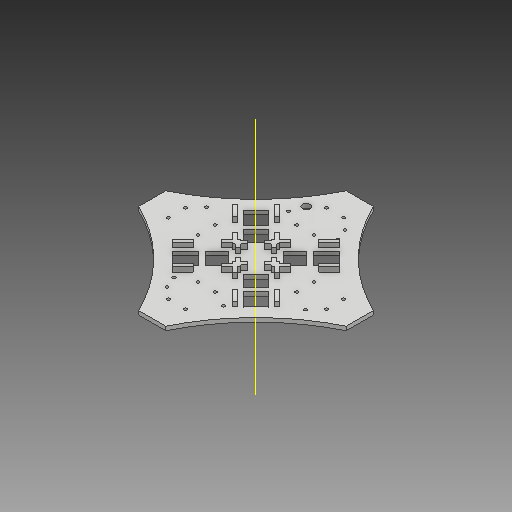
# Autodesk Inventor part: grundplatte_unten
Saved by Autodesk Inventor 2019 (Build 230136000, 136)
## iProperties
Created: 2018-07-23
Part Number: grundplatte_unten
Material: Generisch
Document SubType Name: Modeling
Designer: juliu
Density: 1 g/cm^3
Appearance: Vorgabe
Author: juliu
Autodesk Inventor part; units mm, degrees
ref_plane "YZ Plane" through (0, 0, 0) normal (1, 0, 0) x (0, 1, 0)
ref_plane "XZ Plane" through (0, 0, 0) normal (0, 1, 0) x (-1, 0, 0)
ref_plane "XY Plane" through (0, 0, 0) normal (0, 0, 1) x (1, 0, 0)
sketch "Skizze2" plane through (0, 0, 0) normal (0, 0, 1) x (1, 0, 0)
  line L0 (-268.185, 0) -> (268.185, 0)
  line L1 (0, -270.5283) -> (0, 270.5283) projected
  line L2 (-13.75, 105) -> (13.75, 105)
  line L3 (105, 13.75) -> (105, -13.75)
  line L4 (-105, 13.75) -> (-105, -13.75)
  line L5 (-13.75, -105) -> (13.75, -105)
  arc A0 (-105, 13.75) -> (-13.75, 105) centre (-193.2345, 193.2345) ccw
  arc A1 (13.75, 105) -> (105, 13.75) centre (193.2345, 193.2345) ccw
  arc A2 (105, -13.75) -> (13.75, -105) centre (193.2345, -193.2345) ccw
  arc A3 (-13.75, -105) -> (-105, -13.75) centre (-193.2345, -193.2345) ccw
  point P0 (0, 0)
  dimension "d37" = 105
  dimension "d38" = 27.5
  dimension "d39" = 200
  dimension "d44" = 105
  constraints: 10 end point, 8 point on circle, 4 centre point, 4 symmetric about line, 3 equal length, 3 equal radius, 2 horizontal, 2 vertical, 1 midpoint, 2 other
  measures "d37" distance between parallel lines of L2 L0
  measures "d38" distance of L2.start L2.end
  measures "d39" radius of A0
  measures "d44" distance between parallel lines of L4 L1
extrude "Grundplatte" add sketch "Skizze2" along normal blind 4
sketch "Skizze3" plane through (0, 0, 4) normal (0, 0, 1) x (1, 0, 0)
  line L0 (0, -147) -> (0, 147) projected
  line L1 (13.75, 105) -> (-13.75, 105) projected
  point P0 (0, 0)
  point P1 (-8.75, 80)
  point P2 (-8.75, 50)
  point P3 (8.75, 80)
  point P4 (8.75, 50)
  point P5 (-80, 8.75)
  point P6 (-80, -8.75)
  point P7 (-50, -8.75)
  point P8 (-50, 8.75)
  point P9 (0, 0)
  point P10 (-8.75, -80)
  point P11 (8.75, -80)
  point P12 (8.75, -50)
  point P13 (-8.75, -50)
  point P14 (0, 0)
  point P15 (80, -8.75)
  point P16 (80, 8.75)
  point P17 (50, 8.75)
  point P18 (50, -8.75)
  point P19 (0, 0)
  dimension "d22" = 30
  dimension "d26" = 360
  dimension "d74" = 25
  dimension "d76" = 17.5
  constraints: 2 coincident, 2 symmetric about line, 1 vertical alignment, 19 other
  measures "d22" distance of point (-8.75, 80) point (-8.75, 50)
  measures "d74" distance from line of L1 point (-8.75, 80)
  measures "d76" distance of point (8.75, 50) point (-8.75, 50)
hole "Schrauben Armhalterung" at (-8.75, 80, 4) at (-8.75, 50, 4) at (8.75, 80, 4) at (8.75, 50, 4) at (-80, 8.75, 4) at (-80, -8.75, 4) at (-50, -8.75, 4) at (-50, 8.75, 4) at (-8.75, -80, 4) at (8.75, -80, 4) at (8.75, -50, 4) at (-8.75, -50, 4) at (80, -8.75, 4) at (80, 8.75, 4) at (50, 8.75, 4) at (50, -8.75, 4) direction (0, 0, -1) diameter 3 end through all
sketch "Skizze5" plane through (0, 0, 4) normal (0, 0, 1) x (1, 0, 0)
  line L0 (-7.7782, 20.5061) -> (-19.0919, 31.8198)
  line L1 (-36.0624, 48.7904) -> (-48.7904, 36.0624)
  line L2 (-48.7904, 36.0624) -> (-35.3553, 22.6274)
  line L3 (-20.5061, 7.7782) -> (-7.7782, 20.5061)
  line L4 (147, -147) -> (-147, 147) projected
  line L5 (-19.0919, 31.8198) -> (-31.8198, 19.0919)
  line L6 (-35.3553, 22.6274) -> (-22.6274, 35.3553)
  line L7 (-22.6274, 35.3553) -> (-36.0624, 48.7904)
  line L8 (-20.5061, 7.7782) -> (-31.8198, 19.0919)
  point P0 (0, 0)
  dimension "d49" = 18
  dimension "d50" = 40
  dimension "d71" = 5
  dimension "d72" = 16
  dimension "d73" = 20
  constraints: 16 end point, 6 perpendicular, 3 parallel, 1 point on line, 2 other
  measures "d49" distance of L3.start L0.start
  measures "d50" distance of L1.end L3.start
  measures "d71" distance between parallel lines of L6 L5
  measures "d72" distance between parallel lines of L3 L5
  measures "d73" distance from line of L3 point (0, 0)
extrude "Kühlung Regler" cut sketch "Skizze5" against normal up to next
sketch "Skizze7" plane through (0, 0, 4) normal (0, 0, 1) x (1, 0, 0)
  line L0 (4.2426, 19.799) -> (-5.6569, 29.6985)
  line L1 (-5.6569, 29.6985) -> (-8.4853, 26.8701)
  line L2 (-8.4853, 26.8701) -> (-1.4142, 19.799)
  line L3 (-1.4142, 19.799) -> (-6.364, 14.8492)
  line L4 (-6.364, 14.8492) -> (-3.5355, 12.0208)
  line L5 (4.2426, 19.799) -> (-3.5355, 12.0208)
  line L6 (147, -147) -> (-147, 147) projected
  line L7 (-29.6985, 5.6569) -> (-26.8701, 8.4853)
  line L8 (-26.8701, 8.4853) -> (-19.799, 1.4142)
  line L9 (-19.799, 1.4142) -> (-14.8492, 6.364)
  line L10 (-14.8492, 6.364) -> (-12.0208, 3.5355)
  line L11 (-19.799, -4.2426) -> (-29.6985, 5.6569)
  line L12 (-12.0208, 3.5355) -> (-19.799, -4.2426)
  line L13 (-30.4056, 54.4472) -> (-19.799, 43.8406)
  line L14 (-22.6274, 41.0122) -> (-33.234, 51.6188)
  line L15 (-33.234, 51.6188) -> (-30.4056, 54.4472)
  line L16 (-19.799, 43.8406) -> (-22.6274, 41.0122)
  line L17 (-41.0122, 22.6274) -> (-51.6188, 33.234)
  line L18 (-51.6188, 33.234) -> (-54.4472, 30.4056)
  line L19 (-43.8406, 19.799) -> (-41.0122, 22.6274)
  line L20 (-54.4472, 30.4056) -> (-43.8406, 19.799)
  point P0 (0, 0)
  dimension "d54" = 4
  dimension "d55" = 4
  dimension "d56" = 10
  dimension "d58" = 15
  dimension "d59" = 20
  dimension "d61" = 12
  dimension "d77" = 17
  dimension "d78" = 11
  constraints: 40 end point, 10 symmetric about line, 5 parallel, 4 perpendicular, 2 point on line, 1 collinear, 5 other
  measures "d54" distance of L3.end L4.end
  measures "d55" distance of L0.end L1.end
  measures "d56" distance of L1.end L2.end
  measures "d58" distance of L14.start L14.end
  measures "d59" distance between parallel lines of L1 L16
  measures "d61" distance between parallel lines of L4 L10
  measures "d77" distance between parallel lines of L0 L6
  measures "d78" distance from line of point (0, 0) L5
extrude "Halterung Regler" add sketch "Skizze7" along normal blind 5
pattern_circular "Runde Anordnung1" count 4 over 360 about axis through (0, 0, -10) along (0, 0, 1) of "Halterung Regler"
pattern_circular "Runde Anordnung2" count 4 over 360 about axis through (0, 0, -10) along (0, 0, 1) of "Kühlung Regler"
sketch "Skizze8" plane through (0, 0, 0) normal (0, 0, -1) x (-1, 0, 0)
  line L0 (-17.45, 65) -> (17.45, 65)
  line L1 (17.45, 65) -> (17.45, -65)
  line L2 (17.45, -65) -> (-17.45, -65)
  line L3 (-17.45, -65) -> (-17.45, 65)
  line L4 (0, -147) -> (0, 147) projected
  line L5 (147, 0) -> (-147, 0) projected
  point P0 (0, 0)
  point P1 (-25, 58)
  point P2 (25, 58)
  point P3 (-25, -58)
  point P4 (25, -58)
  dimension "d39" = 200
  dimension "d79" = 130
  dimension "d80" = 34.9
  dimension "d81" = 7
  dimension "d82" = 50
  constraints: 8 end point, 3 symmetric about line, 2 parallel, 1 horizontal, 1 perpendicular, 2 other
  measures "d79" distance of L0.end L1.end
  measures "d80" distance of L0.start L0.end
  measures "d81" distance from line of L0 point (25, 58)
  measures "d82" distance of point (-25, 58) point (25, 58)
hole "Schrauben Akkuhalter" at (25, 58, 0) at (-25, 58, 0) at (-25, -58, 0) at (25, -58, 0) direction (0, 0, 1) diameter 3 end through all
sketch "Skizze9" plane through (0, 0, 0) normal (0, 0, -1) x (-1, 0, 0)
  line L0 (0, -147) -> (0, 147) projected
  line L1 (147, 0) -> (-147, 0) projected
  circle A0 centre (25, 58) radius 1.5 projected
  point P0 (0, 0)
  point P1 (20, 71)
  dimension "d39" = 200
  dimension "d90" = 20
  dimension "d91" = 13
  measures "d90" distance from line of L0 point (20, 71)
  measures "d91" vertical distance of A0.centre point (20, 71)
hole "Kabel Akku" at (-20, 71, 0) direction (0, 0, 1) diameter 8 end through all
sketch "Skizze11" plane through (0, 0, 0) normal (0, 0, -1) x (-1, 0, 0)
  line L0 (147, 0) -> (-147, 0) projected
  line L1 (0, -147) -> (0, 147) projected
  line L2 (-13.75, -105) -> (13.75, -105) projected
  point P0 (0, 0)
  point P1 (20, -70)
  dimension "d39" = 200
  dimension "d108" = 20
  dimension "d109" = 35
  measures "d108" distance from line of L1 point (20, -70)
  measures "d109" distance from line of L2 point (20, -70)
hole "Schrauben Kuppel" at (-20, -70, 0) direction (0, 0, 1) diameter 3 end through all
pattern_circular "Runde Anordnung3" count 4 over 360 about axis through (0, 0, -10) along (0, 0, 1) of "Schrauben Kuppel"
